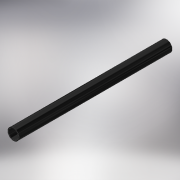
# Autodesk Inventor part: Tube0
Saved by Autodesk Inventor 2018 (Build 220112000, 112)
## iProperties
Created: 2018-11-08
Part Number: Tube0
Material: ABS Plastic
Document SubType Name: Modeling
Designer: Isaac Newcomb
Density: 1.06 g/cm^3
Appearance: Smooth - White
Diameter: 10.000 mm
Wallthickness: 0.600 mm
TuningPlugLength: 12.000 mm
Author: Isaac Newcomb
Autodesk Inventor part; units mm, degrees
ref_plane "YZ Plane" through (0, 0, 0) normal (1, 0, 0) x (0, 1, 0)
ref_plane "XZ Plane" through (0, 0, 0) normal (0, 1, 0) x (-1, 0, 0)
ref_plane "XY Plane" through (0, 0, 0) normal (0, 0, 1) x (1, 0, 0)
sketch "Circles" plane through (0, 0, 0) normal (0, 0, 1) x (1, 0, 0)
  circle A0 centre (0, 0) radius 5
  circle A1 centre (0, 0) radius 4.4
  dimension "Diameter" = 10
  dimension "Wallthickness" = 0.6
  constraints: 2 centre point, 2 coincident
  measures "Diameter" diameter of A0
  measures "Wallthickness" radial gap between concentric circles of A1 A0
extrude "Tube" add sketch "Circles" along normal blind 134
equation "\"Length\" = CalculatedLength"
equation "\"DesiredCavityLength\" = 163"
equation "\"PostValveExtraLength\" = WhistleHousingLength - TubeSocketLength"
equation "\"TuningPlugLength\" = 12"
equation "\"CalculatedLength\" = TuningPlugLength + DesiredCavityLength - PostValveExtraLength"
equation "\"WhistleHousingLength\" = 51"
equation "\"TubeSocketLength\" = 10"
body "Solid1"
